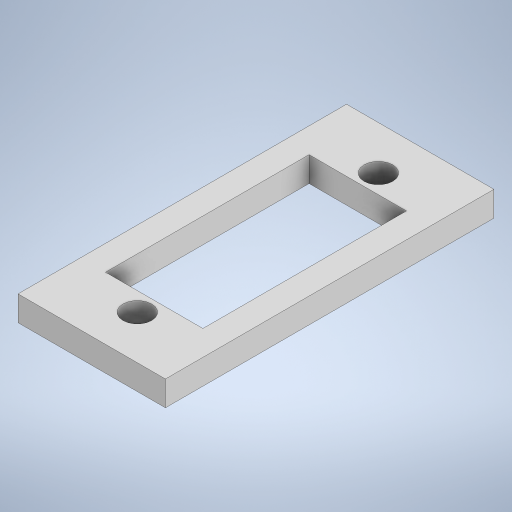
# Autodesk Inventor part: SwitchTest
Saved by Autodesk Inventor 2024.2 (Build 282272000, 272)
## iProperties
Created: 2024-04-18
Part Number: SwitchTest
Material: Generic
Document SubType Name: Modeling
Designer: ringl
Density: 1 g/cm^3
Appearance: Default
Author: ringl
Autodesk Inventor part; units mm, degrees
ref_plane "YZ Plane" through (0, 0, 0) normal (1, 0, 0) x (0, 1, 0)
ref_plane "XZ Plane" through (0, 0, 0) normal (0, 1, 0) x (-1, 0, 0)
ref_plane "XY Plane" through (0, 0, 0) normal (0, 0, 1) x (1, 0, 0)
sketch "Sketch1" plane through (0, 0, 0) normal (0, 1, 0) x (-1, 0, 0)
  line L0 (0, 0) -> (7.8, 0)
  line L1 (7.8, 0) -> (7.8, -16.3)
  line L2 (7.8, -16.3) -> (0, -16.3)
  line L3 (0, -16.3) -> (0, 0)
  line L4 (9.8, -21.3) -> (-2, -21.3)
  line L5 (-2, -21.3) -> (-2, 5)
  line L6 (-2, 5) -> (9.8, 5)
  line L7 (9.8, 5) -> (9.8, -21.3)
  circle A0 centre (3.75, 1.5) radius 1.15
  circle A1 centre (3.75, -17.8) radius 1.15
  dimension "d0" = 7.8
  dimension "d1" = 16.3
  dimension "d2" = 2
  dimension "d3" = 2
  dimension "d4" = 5
  dimension "d5" = 5
  dimension "d6" = 2.3
  dimension "d7" = 2.3
  dimension "d8" = 1.5
  dimension "d9" = 1.5
  dimension "d10" = 3.75
  constraints: 16 end point, 4 parallel, 2 centre point, 2 horizontal, 2 perpendicular, 1 vertical alignment
  measures "d0" distance of L1.end L2.end
  measures "d1" distance of L0.end L1.end
  measures "d2" distance between parallel lines of L3 L5
  measures "d3" distance between parallel lines of L7 L1
  measures "d4" distance between parallel lines of L0 L6
  measures "d5" distance between parallel lines of L4 L2
  measures "d6" diameter of A0
  measures "d7" diameter of A1
  measures "d8" distance from line of L0 A0.centre
  measures "d9" distance from line of L2 A1.centre
  measures "d10" distance from line of A1.centre L3
extrude "Extrusion1" add sketch "Sketch1" along normal blind 2
body "Solid1"
